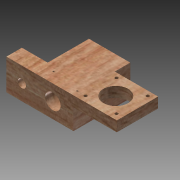
# Autodesk Inventor part: X_Top_MotorSide_V3
Saved by Autodesk Inventor 2014 (Build 180170000, 170)
## iProperties
Created: 2013-12-13
Part Number: X_Top_MotorSide_V3
Material: Birch
Document SubType Name: Modeling
Designer: Bram
Density: 0.512 g/cm^3
Appearance: Birch - Natural Medium Gloss
Author: Bram
Autodesk Inventor part; units mm, degrees
ref_plane "YZ Plane" through (0, 0, 0) normal (1, 0, 0) x (0, 1, 0)
ref_plane "XZ Plane" through (0, 0, 0) normal (0, 1, 0) x (-1, 0, 0)
ref_plane "XY Plane" through (0, 0, 0) normal (0, 0, 1) x (1, 0, 0)
sketch "Sketch1" plane through (0, 0, 0) normal (0, 1, 0) x (-1, 0, 0)
  line L0 (0, 0) -> (107, 0)
  line L1 (107, 0) -> (107, 30)
  line L2 (107, 30) -> (42, 30)
  line L3 (0, 20) -> (0, 0)
  line L4 (42, 30) -> (42, 20)
  line L5 (42, 20) -> (0, 20)
  circle A0 centre (62, 15) radius 7.5
  circle A1 centre (92, 15) radius 4
  dimension "d6" = 15
  dimension "d7" = 8
  constraints: 12 end point, 2 centre point, 2 parallel, 1 horizontal, 1 perpendicular
  measures "d6" diameter of A0
  measures "d7" diameter of A1
extrude "Extrusion1" add sketch "Sketch1" along normal blind 55
sketch "Sketch2" plane through (-107, 0, 30) normal (0, 0, 1) x (1, 0, 0)
  line L0 (0, 55) -> (25, 55)
  line L1 (25, 55) -> (25, 15)
  line L2 (25, 15) -> (0, 15)
  line L3 (0, 15) -> (0, 55)
  point P0 (107, 0)
  dimension "d10" = 25
  dimension "d11" = 40
  constraints: 8 end point, 2 parallel, 1 horizontal, 1 perpendicular
  measures "d10" distance of L1.end L2.end
  measures "d11" distance of L0.end L1.end
extrude "Extrusion2" cut sketch "Sketch2" against normal blind 55
sketch "Sketch3" plane through (-42, 0, 20) normal (0, 0, 1) x (1, 0, 0)
  line L0 (0, 55) -> (42, 55)
  line L1 (42, 55) -> (42, 40)
  line L2 (42, 40) -> (0, 40)
  line L3 (0, 40) -> (0, 55)
  circle A0 centre (21, 20) radius 12
  circle A1 centre (6.2237, 35.5013) radius 1.5
  circle A2 centre (36.5, 35.5) radius 1.5
  circle A3 centre (36.2237, 5.5013) radius 1.5
  circle A4 centre (6.2237, 5.5013) radius 1.5
  dimension "d14" = 42
  dimension "d15" = 15
  dimension "d16" = 24
  dimension "d22" = 3
  dimension "d23" = 3
  dimension "d24" = 3
  dimension "d25" = 3
  constraints: 8 end point, 5 centre point, 2 parallel, 1 horizontal, 1 perpendicular
  measures "d14" distance of L1.end L2.end
  measures "d15" distance of L0.end L1.end
  measures "d16" diameter of A0
  measures "d22" diameter of A1
  measures "d23" diameter of A2
  measures "d24" diameter of A3
  measures "d25" diameter of A4
extrude "Extrusion3" cut sketch "Sketch3" against normal blind 55
sketch "Sketch4" plane through (-42, 0, 20) normal (0, 0, 1) x (1, 0, 0)
  line L0 (42, 40) -> (0, 40) projected
  line L1 (0, 0) -> (0, 40) projected
  line L2 (0, 0) -> (42, 0) projected
  line L3 (42, 0) -> (42, 40) projected
  circle A0 centre (21, 20) radius 12 projected
  circle A1 centre (36.2237, 5.5013) radius 1.5 projected
  circle A2 centre (6.2237, 35.5013) radius 1.5 projected
  circle A3 centre (36.5, 35.5) radius 1.5 projected
  circle A4 centre (6.2237, 5.5013) radius 1.5 projected
extrude "Extrusion4" add sketch "Sketch4" along normal blind 10
sketch "Sketch5" plane through (0, 0, 0) normal (0, 0, -1) x (-1, 0, 0)
  line L0 (42, 40) -> (0, 40) projected
  line L1 (0, 0) -> (0, 40) projected
  line L2 (0, 0) -> (107, 0) projected
  circle A0 centre (35.7763, 5.5013) radius 1.5 projected
  circle A1 centre (5.5, 35.5) radius 1.5 projected
  circle A2 centre (35.7763, 35.5013) radius 1.5 projected
  circle A3 centre (5.7763, 5.5013) radius 1.5 projected
  circle A4 centre (21, 20) radius 12 projected
  line L3 (42, 40) -> (42, 0)
  constraints: 2 end point, 1 perpendicular, 1 point on line
extrude "Extrusion5" cut sketch "Sketch5" against normal blind 20
body "Solid1"
